Bielle (Autodesk Fusion 360 design; units mm, degrees)
Autodesk Fusion 360 part; units mm, degrees
note: some values were not read from the file. Set by a fixed rule: which sketch regions a step uses.
sketch "Sketch1" plane through (0, 0, 0) normal (0, 0, 1) x (1, 0, 0)
  circle A0 centre (0, 0) radius 18 construction
  line L0 (-3.7812, 75.9244) -> (-17.6785, 3.387)
  circle A1 centre (0, 75.2) radius 3.85 construction
  circle A2 centre (0, 0) radius 19.5
  line L1 (17.6785, 3.387) -> (3.7812, 75.9244)
  line L2 (0, 0) -> (0, 100) construction
  circle A3 centre (0, 75.2) radius 8.6
  circle A4 centre (0, 0) radius 11.1
  circle A5 centre (0, 0) radius 5.25
  dimension "d2" = 39
  dimension "d3" = 36
  dimension "d4" = 7.7
  dimension "d5" = 75.2
  dimension "d15" = 22.2
  dimension "d16" = 10.5
  constraint coincident L0.end A0
  constraint coincident L0.start A1
  constraint coincident A0.centre A2.centre
  constraint coincident A0 L1.start
  constraint coincident A1 L1.end
  constraint tangent A1 L1
  constraint tangent A0 L1
  constraint tangent A0 L0
  constraint tangent L0 A1
  constraint vertical L2
  constraint coincident A1.centre L2
  measures "d2" diameter of A2
  measures "d3" diameter of A0
  measures "d4" diameter of A1
  measures "d5" distance of A0.centre A1.centre
  measures "d15" diameter of A4
  measures "d16" diameter of A5
extrude "Extrude1" add sketch "Sketch1" along normal blind 13 contours L0 A2 L1 A3 | A3 | A2
extrude "Extrude4" add sketch "Sketch1" along normal blind 6 contours A4
extrude "Extrude5" add sketch "Sketch1" along normal blind 4 contours L0 A2 L1 A3
fillet "Fillet2" radius 20 2 edges at (-5.2282, 68.3717, 6.5) (5.2282, 68.3717, 6.5)
sketch "Sketch2" plane through (0, 0, 0) normal (0, 0, -1) x (1, 0, 0)
  arc A0 (6.7512, -60.4223) -> (7.9367, -71.888) centre (26.394, -64.1856) ccw
  line L0 (6.7512, -60.4223) -> (16.2672, -10.753)
  arc A1 (16.2672, -10.753) -> (-16.2672, -10.753) centre (0, 0) ccw
  line L1 (-16.2672, -10.753) -> (-6.7512, -60.4223)
  arc A2 (-7.9367, -71.888) -> (-6.7512, -60.4223) centre (-26.394, -64.1856) ccw
  arc A3 (-7.9367, -71.888) -> (7.9367, -71.888) centre (0, -75.2) ccw
  circle A4 centre (0, 0) radius 16.75
  circle A5 centre (0, 0) radius 5.25
  circle A6 centre (0, 0) radius 4.5
  dimension "d27" = 33.5
  constraint coincident A1.centre A4.centre
  constraint concentric A4 A6
  measures "d27" diameter of A4
extrude "Extrude6" add sketch "Sketch2" along normal blind 11 contours A4
sketch "Sketch3" plane through (0, 0, -11) normal (0, 0, -1) x (1, 0, 0)
  circle A0 centre (0, 0) radius 5.25
  circle A1 centre (0, 0) radius 16.75
  line L0 (10, 5.7735) -> (0, 11.547)
  line L1 (0, 11.547) -> (-10, 5.7735)
  line L2 (-10, 5.7735) -> (-10, -5.7735)
  line L3 (-10, -5.7735) -> (0, -11.547)
  line L4 (0, -11.547) -> (10, -5.7735)
  line L5 (10, -5.7735) -> (10, 5.7735)
  constraint coincident A0.centre A1.centre
extrude "Extrude7" add sketch "Sketch3" along normal blind 10 contours L0 L1 L2 L3 L4 L5
sketch "Sketch4" plane through (0, 0, 0) normal (0, 0, -1) x (1, 0, 0)
  circle A0 centre (0, 0) radius 16.75
  arc A1 (6.7512, -60.4223) -> (7.9367, -71.888) centre (26.394, -64.1856) ccw
  line L0 (6.7512, -60.4223) -> (16.2672, -10.753)
  arc A2 (16.2672, -10.753) -> (-16.2672, -10.753) centre (0, 0) ccw
  line L1 (-16.2672, -10.753) -> (-6.7512, -60.4223)
  arc A3 (-7.9367, -71.888) -> (-6.7512, -60.4223) centre (-26.394, -64.1856) ccw
  arc A4 (-7.9367, -71.888) -> (7.9367, -71.888) centre (0, -75.2) ccw
  circle A5 centre (0, -75.2) radius 6.55
  circle A6 centre (0, -75.2) radius 5
  dimension "d32" = 13.1
  dimension "d33" = 10
  constraint concentric A4 A5
  constraint concentric A5 A6
  measures "d32" diameter of A5
  measures "d33" diameter of A6
extrude "Extrude8" cut sketch "Sketch4" against normal through all contours A6
extrude "Extrude9" cut sketch "Sketch4" against normal blind 9 contours A5
sketch "Sketch5" plane through (0, 0, 6) normal (0, 0, 1) x (-1, 0, 0)
  circle A0 centre (0, 0) radius 5.25
  circle A1 centre (0, 0) radius 11.1
  circle A2 centre (0, 0) radius 6.5
  dimension "d37" = 13
  constraint concentric A0 A2
  measures "d37" diameter of A2
extrude "Extrude10" cut sketch "Sketch5" against normal blind 1 contours A2
equation "d20 = 13 mm - 7 mm"
equation "d22 = ( ( 13 / 2 ) * 1 mm ) - 2.5 mm"
